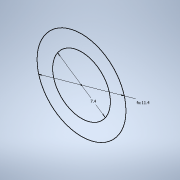
# Autodesk Inventor part: Part6
Saved by Autodesk Inventor 2022 (Build 260153000, 153)
## iProperties
Created: 2021-09-14
Part Number: Part6
Material: Generic
Document SubType Name: Modeling
Designer: tecware
Density: 1 g/cm^3
Appearance: Default
Author: tecware
Autodesk Inventor part; units mm, degrees
ref_plane "XY Plane" through (0, 0, 0) normal (0, 0, 1) x (1, 0, 0)
sketch "Sketch1" plane through (0, 0, 0) normal (0, 0, 1) x (1, 0, 0)
  circle A0 centre (0, 0) radius 3.7
  circle A1 centre (0, 0) radius 5.7
  dimension "d0" = 7.4
  dimension "d1" = 11.4
  constraints: 2 centre point, 2 coincident
  measures "d0" diameter of A0
  measures "d1" diameter of A1
extrude "Extrusion1" add sketch "Sketch1" along normal mid plane 30
ref_plane "Work Plane1" through (0, 5.7, 0) normal (0, 1, 0) x (-1, 0, 0)
ref_plane "Work Plane2" through (-5.7, 0, 0) normal (1, 0, 0) x (0, 1, 0)
sketch "Sketch2" plane through (-5.7, 5.7, 0) normal (1, 0, 0) x (0, 1, 0)
  point P0 (-5.7, 0)
  point P1 (-5.7, 0)
  constraints: 1 coincident
hole "Hole1" at (-5.7, 0, 0) direction (1, 0, 0) diameter 2 depth 3
ref_plane "Work Plane4" through (30.7, 0, 0) normal (1, 0, 0) x (0, 1, 0)
ref_plane "Work Plane3" through (5.7, 0, 0) normal (1, 0, 0) x (0, 1, 0)
sketch "Sketch4" plane through (30.7, 0, 0) normal (1, 0, 0) x (0, 1, 0)
  circle A0 centre (0, 0) radius 5.7
  circle A1 centre (0, 0) radius 3.7
  dimension "d19" = 7.4
  dimension "d20" = 11.4
  constraints: 2 centre point, 2 coincident
  measures "d19" diameter of A1
  measures "d20" diameter of A0
extrude "Extrusion3" add sketch "Sketch4" against normal up to surface contours A0 | A1 round surface about axis through (0, 0, 0) along (0, 0, 1) radius 5.7 far side no
sketch "Sketch5" plane through (30.7, 0, 0) normal (1, 0, 0) x (0, 1, 0)
  circle A0 centre (0, 0) radius 5.7
  circle A1 centre (0, 0) radius 3.7
  dimension "d23" = 7.4
  dimension "d24" = 11.4
  constraints: 2 centre point, 2 coincident
  measures "d23" diameter of A1
  measures "d24" diameter of A0
extrude "Extrusion4" cut sketch "Sketch5" against normal up to surface contours A1 round surface about axis through (0, 0, 0) along (0, 0, 1) radius 3.7 far side no
sketch "Sketch6" plane through (0, 5.7, 0) normal (0, 1, 0) x (-1, 0, 0)
  line L0 (0, 0) -> (-31, 0) construction
  point P0 (-15.5, 0)
  constraints: 2 end point, 1 horizontal, 1 midpoint
hole "Hole2" at (15.5, 5.7, 0) direction (0, -1, 0) diameter 2 depth 3
equation "\"d25\" = d24"
body "Solid1"
